Autodesk Inventor part; units mm, degrees
(part 3 of 9)
sketch "Sketch24" plane through (0, 0, 0) normal (1, 0, 0) x (0, 0, -1)
  circle A0 centre (-187.1176, -166.8269) radius 2.4892 projected
  circle A1 centre (-174.2102, -166.8866) radius 2.4892 projected
  circle A2 centre (-167.2175, -120.5501) radius 2.4892 projected
  circle A3 centre (-180.1195, -116.9252) radius 2.4892 projected
  circle A4 centre (-193.0957, -120.1058) radius 2.4892 projected
  circle A5 centre (-186.8225, -117.6771) radius 2.4892 projected
  circle A6 centre (-173.4354, -117.9041) radius 2.4892 projected
  circle A7 centre (-168.1768, -164.3742) radius 2.4892 projected
  circle A8 centre (-180.6733, -167.7222) radius 2.4892 projected
  circle A9 centre (-193.0957, -164.2646) radius 2.4892 projected
  circle A10 centre (0, 0) radius 13.335 projected
  circle A11 centre (160.7915, -118.9794) radius 2.5527 projected
  line L0 (182.8723, -109.8807) -> (181.7836, -109.2266) projected
  arc A12 (170.0112, -99.2275) -> (190.7761, 48.5222) centre (0, 0) ccw projected
  line L1 (204.8485, 54.889) -> (206.0753, 55.2177) projected
  arc A13 (175.4872, -102.4426) -> (196.9261, 50.1033) centre (0, 0) ccw projected
  arc A14 (159.1231, -92.6879) -> (178.5072, 45.237) centre (0, 0) ccw projected
  line L2 (180.312, 48.3145) -> (181.5388, 48.6432) projected
  arc A15 (164.6013, -95.8992) -> (184.6584, 46.8139) centre (0, 0) ccw projected
  line L3 (161.0985, -96.7977) -> (160.0098, -96.1436) projected
  arc A16 (180.8991, -105.7674) -> (203.0448, 51.8076) centre (0, 0) ccw projected
  line L4 (192.5803, 51.6017) -> (193.8071, 51.9305) projected
  arc A17 (186.3731, -108.9857) -> (209.1938, 53.3924) centre (0, 0) ccw projected
  line L5 (171.9854, -103.3393) -> (170.8967, -102.6851) projected
  circle A18 centre (239.2356, -31.496) radius 3.3782 projected
  circle A19 centre (223.7295, 90.3926) radius 3.3782 projected
  circle A20 centre (239.2356, 31.496) radius 3.3782 projected
  circle A21 centre (221.404, -95.9477) radius 3.3782 projected
  line L6 (-35.2916, -50.8) -> (42.0514, -50.8) projected
  arc A22 (74.705, -62.6849) -> (42.0514, -50.8) centre (42.0514, -101.6) ccw projected
  line L7 (74.705, -62.6849) -> (143.4787, -120.3929) projected
  arc A23 (143.8351, -124.9069) -> (143.4787, -120.3929) centre (141.4378, -122.8251) ccw projected
  arc A24 (141.8978, -127.1034) -> (143.8351, -124.9069) centre (0, 0) ccw projected
  arc A25 (141.8978, -127.1034) -> (141.494, -128.2246) centre (143.0803, -128.1626) ccw projected
  line L8 (141.6194, -131.4328) -> (141.494, -128.2246) projected
  arc A26 (141.6194, -131.4328) -> (142.123, -132.5318) centre (143.2057, -131.3708) ccw projected
  line L9 (142.123, -132.5318) -> (176.2311, -164.3381) projected
  arc A27 (176.2311, -164.3381) -> (194.6236, -163.2104) centre (184.8924, -155.0499) ccw projected
  arc A28 (194.6236, -163.2104) -> (235.5329, 95.0804) centre (0, 0) ccw projected
  arc A29 (235.5329, 95.0804) -> (218.389, 101.8364) centre (223.7562, 90.3263) ccw projected
  line L10 (218.389, 101.8364) -> (173.6183, 80.9596) projected
  arc A30 (152.1493, 76.2) -> (173.6183, 80.9596) centre (152.1493, 127) ccw projected
  line L11 (152.1493, 76.2) -> (-101.6, 76.2) projected
  line L12 (-101.6, 76.2) -> (-199.482, -21.682) projected
  line L13 (-199.482, -21.682) -> (-199.482, -255.599) projected
  line L14 (-199.482, -255.599) -> (-35.2916, -255.599) projected
  line L15 (-35.2916, -255.599) -> (-35.2916, -50.8) projected
  line L16 (149.831, -89.2272) -> (89.9434, -38.9755) projected
  line L17 (88.9, -36.7379) -> (88.9, -15.621) projected
  line L18 (91.821, -12.7) -> (174.1799, -12.7) projected
  arc A31 (154.2425, -88.4425) -> (177.0893, -15.8819) centre (0, 0) ccw projected
  line L19 (88.9, -0.254) -> (88.9, 0.254) projected
  line L20 (91.821, 3.175) -> (174.4218, 3.175) projected
  line L21 (177.3428, 0.254) -> (177.3428, -0.254) projected
  line L22 (174.4218, -3.175) -> (91.821, -3.175) projected
  arc A32 (177.0893, 15.8819) -> (169.6939, 53.0738) centre (0, 0) ccw projected
  line L23 (174.1799, 12.7) -> (91.821, 12.7) projected
  line L24 (88.9, 15.621) -> (88.9, 17.1891) projected
  line L25 (90.5865, 19.8364) -> (165.6716, 54.8492) projected
  circle A33 centre (-80.2428, -88.2574) radius 2.4892 projected
  circle A34 centre (-101.8395, -100.8579) radius 2.4892 projected
  circle A35 centre (-93.0185, -51.5569) radius 2.4892 projected
  circle A36 centre (-93.2858, -99.3592) radius 2.4892 projected
  circle A37 centre (-110.6604, -51.6228) radius 2.4892 projected
  circle A38 centre (-124.2369, -62.8574) radius 2.4892 projected
  circle A39 centre (-101.8395, -50.0579) radius 2.4892 projected
  circle A40 centre (-110.3931, -99.2933) radius 2.4892 projected
  circle A41 centre (-85.7798, -94.9817) radius 2.4892 projected
  arc A42 (174.1799, 12.7) -> (177.0893, 15.8819) centre (174.1799, 15.621) ccw projected
  arc A43 (88.9, 15.621) -> (91.821, 12.7) centre (91.821, 15.621) ccw projected
  arc A44 (90.5865, 19.8364) -> (88.9, 17.1891) centre (91.821, 17.1891) ccw projected
  arc A45 (169.6939, 53.0738) -> (165.6716, 54.8492) centre (166.9061, 52.2019) ccw projected
  arc A46 (91.821, 3.175) -> (88.9, 0.254) centre (91.821, 0.254) ccw projected
  arc A47 (177.3428, 0.254) -> (174.4218, 3.175) centre (174.4218, 0.254) ccw projected
  arc A48 (174.4218, -3.175) -> (177.3428, -0.254) centre (174.4218, -0.254) ccw projected
  arc A49 (88.9, -0.254) -> (91.821, -3.175) centre (91.821, -0.254) ccw projected
  arc A50 (88.9, -36.7379) -> (89.9434, -38.9755) centre (91.821, -36.7379) ccw projected
  arc A51 (91.821, -12.7) -> (88.9, -15.621) centre (91.821, -15.621) ccw projected
  arc A52 (177.0893, -15.8819) -> (174.1799, -12.7) centre (174.1799, -15.621) ccw projected
  arc A53 (149.831, -89.2272) -> (154.2425, -88.4425) centre (151.7086, -86.9895) ccw projected
  arc A54 (170.0112, -99.2275) -> (170.8967, -102.6851) centre (172.2049, -100.5079) ccw projected
  arc A55 (192.5803, 51.6017) -> (190.7761, 48.5222) centre (193.2377, 49.1483) ccw projected
  arc A56 (196.9261, 50.1033) -> (193.8071, 51.9305) centre (194.4645, 49.477) ccw projected
  arc A57 (171.9854, -103.3393) -> (175.4872, -102.4426) centre (173.2936, -101.1621) ccw projected
  arc A58 (180.312, 48.3145) -> (178.5072, 45.237) centre (180.9694, 45.861) ccw projected
  arc A59 (184.6584, 46.8139) -> (181.5388, 48.6432) centre (182.1962, 46.1897) ccw projected
  arc A60 (161.0985, -96.7977) -> (164.6013, -95.8992) centre (162.4067, -94.6205) ccw projected
  arc A61 (159.1231, -92.6879) -> (160.0098, -96.1436) centre (161.3179, -93.9664) ccw projected
  arc A62 (204.8485, 54.889) -> (203.0448, 51.8076) centre (205.5059, 52.4355) ccw projected
  arc A63 (209.1938, 53.3924) -> (206.0753, 55.2177) centre (206.7327, 52.7643) ccw projected
  arc A64 (182.8723, -109.8807) -> (186.3731, -108.9857) centre (184.1805, -107.7035) ccw projected
  arc A65 (180.8991, -105.7674) -> (181.7836, -109.2266) centre (183.0918, -107.0494) ccw projected
  arc A66 (-99.6119, -84.758) -> (-99.4903, -84.728) centre (-101.8395, -75.4579) ccw projected
  arc A67 (-99.4903, -84.728) -> (-104.0551, -66.155) centre (-101.7058, -75.4251) ccw projected
  arc A68 (-99.7334, -84.7881) -> (-99.6119, -84.758) centre (-101.9731, -75.491) ccw projected
  arc A69 (-99.8547, -84.8183) -> (-99.7334, -84.7881) centre (-102.1066, -75.5241) ccw projected
  arc A70 (-104.4917, -66.2632) -> (-99.8547, -84.8183) centre (-102.2399, -75.5574) ccw projected
  arc A71 (-104.3463, -66.227) -> (-104.4917, -66.2632) centre (-102.1066, -75.5241) ccw projected
  arc A72 (-104.2008, -66.1909) -> (-104.3463, -66.227) centre (-101.9731, -75.491) ccw projected
  arc A73 (-104.0551, -66.155) -> (-104.2008, -66.1909) centre (-101.8395, -75.4579) ccw projected
  circle A74 centre (0, 0) radius 14.2875
  circle A75 centre (-101.8395, -75.4579) radius 31.75
  line L26 (-136.6187, 12.3445) -> (-98.9084, -11.187)
  line L27 (-98.9084, -11.187) -> (-75.3768, 26.5234)
  line L28 (-75.3768, 26.5234) -> (-113.0872, 50.0549)
  line L29 (-113.0872, 50.0549) -> (-136.6187, 12.3445)
  line L30 (-136.6187, 12.3445) -> (-75.3768, 26.5234) construction
  line L31 (-98.9084, -11.187) -> (-113.0872, 50.0549) construction
  circle A76 centre (-101.8395, -75.4579) radius 44.565
  circle A77 centre (0, 0) radius 15.915
  line L32 (-119.5903, -34.5807) -> (-6.3391, 14.598)
  line L33 (-67.9013, -104.3411) -> (12.12, -10.3147)
  circle A78 centre (0, 0) radius 47.752
  line L34 (-107.8805, 35.2378) -> (-5.6488, 47.4167)
  circle A79 centre (-105.9978, 19.434) radius 15.9156
  line L35 (-113.3646, 5.3259) -> (-22.1029, -42.3286)
  line L36 (-100.8386, 14.2238) -> (-107.9303, 12.3609)
  line L37 (-107.9303, 12.3609) -> (-113.0895, 17.571)
  line L38 (-113.0895, 17.571) -> (-111.157, 24.6441)
  line L39 (-111.157, 24.6441) -> (-104.0652, 26.507)
  line L40 (-104.0652, 26.507) -> (-98.906, 21.2969)
  line L41 (-98.906, 21.2969) -> (-100.8386, 14.2238)
  circle A80 centre (-105.9978, 19.434) radius 7.3323
  circle A81 centre (-101.8395, -75.4579) radius 9.5631
  circle A82 centre (-105.9978, 19.434) radius 9.5631
  circle A83 centre (-101.8395, -75.4579) radius 25.4
  circle A84 centre (-105.9978, 19.434) radius 25.4
  line L42 (-101.8395, -75.4579) -> (0, 0)
  circle A85 centre (0, 0) radius 50.8
  circle A86 centre (-105.9978, 19.434) radius 31.4309
  arc A87 (136.2027, -114.2876) -> (161.1415, 75.1415) centre (0, 0) ccw
  line L43 (0, 0) -> (136.2027, -114.2876)
  line L44 (0, 0) -> (146.4464, 0)
  circle A88 centre (33.8645, -135.5333) radius 88.9
  circle A89 centre (-76.4174, -178.6042) radius 25.4
  line L45 (-88.4199, -21.0451) -> (-93.4785, -9.396)
  circle A90 centre (-76.4174, -178.6042) radius 21.4859
  line L46 (-141.7593, -95.2683) -> (-95.6637, -188.1553)
  line L47 (-57.286, -74.4485) -> (-54.9371, -178.1175)
  line L48 (136.2027, -114.2876) -> (90.5518, -239.7125)
  circle A91 centre (31.6927, -141.5004) radius 88.9
  line L49 (-52.5492, -187.2916) -> (90.6599, -239.4154)
  line L50 (-105.9978, 19.434) -> (0, 0)
  line L51 (-76.4174, -204.0042) -> (-76.4174, -178.6042)
  line L52 (136.2027, -114.2876) -> (136.2027, -239.7125)
  line L53 (-58.8554, 19.434) -> (-105.9978, 19.434)
  circle A92 centre (-17.4502, -276.5193) radius 88.9
  line L54 (-501.4434, -455.6125) -> (248.5176, -455.6125)
  line L55 (-550.7161, -581.025) -> (328.0098, -581.025)
  circle A93 centre (-54.61, -366.7125) radius 88.9
  line L56 (-54.61, -280.9875) -> (-16.51, -280.9875)
  line L57 (-16.51, -280.9875) -> (-16.51, -363.5375)
  line L58 (-16.51, -363.5375) -> (-54.61, -363.5375)
  line L59 (-54.61, -363.5375) -> (-54.61, -280.9875)
  line L60 (-54.61, -322.2625) -> (-16.51, -322.2625)
  line L61 (-54.61, -366.7125) -> (-54.61, -277.8125)
  circle A94 centre (-16.51, -277.8125) radius 88.9
  line L62 (-16.51, -277.8125) -> (-16.51, -366.7125)
  circle A95 centre (-180.2765, -142.3655) radius 31.75
  circle A96 centre (-180.2765, -142.3655) radius 25.4
  circle A97 centre (-180.2765, -142.3655) radius 44.563
  circle A98 centre (-180.2765, -142.3655) radius 9.5631
  line L63 (-194.9575, -184.4408) -> (-91.0984, -220.6795)
  line L64 (-165.5955, -100.2902) -> (-61.7364, -136.5289)
  circle A99 centre (-76.4174, -178.6042) radius 44.563
  line L65 (-167.0299, -113.5109) -> (-119.1112, -9.1307)
  line L66 (-156.1209, -121.7605) -> (-135.7449, -104.3796)
  circle A100 centre (29.8359, -136.4768) radius 88.9
  line L67 (-116.4833, -117.4265) -> (-112.2994, -105.4355)
  point P0 (-35.56, -322.2625)
  dimension "d735" = 63.5
  dimension "d734" = 28.575
  dimension "d736" = 44.45
  dimension "d737" = 31.83
  dimension "d738" = 89.13
  dimension "d739" = 95.504
  dimension "d740" = 31.8313
  dimension "d741" = 12.7
  dimension "d742" = 19.1262
  dimension "d743" = 19.1262
  dimension "d744" = 50.8
  dimension "d745" = 50.8
  dimension "d746" = 107.7646
  dimension "d747" = 126.7485
  dimension "d748" = 101.6
  dimension "d749" = 127
  dimension "d750" = 40
  dimension "d751" = 177.8
  dimension "d752" = 50.8
  dimension "d753" = 12.7
  dimension "d754" = 6.35
  dimension "d755" = 106.233
  dimension "d756" = 152.4
  dimension "d757" = 279.1458
  dimension "d758" = 25
  dimension "d759" = 20
  dimension "d760" = 47.1424
  dimension "d761" = 42.9717
  dimension "d762" = 125.4125
  dimension "d763" = 656.1665
  dimension "d764" = 82.55
  dimension "d765" = 38.1
  dimension "d766" = 1.5989
  dimension "d767" = 35.56
  dimension "d768" = 215.9
  dimension "d769" = 215.9
  dimension "d770" = 26.7819
  dimension "d771" = 114.8539
  dimension "d772" = 109.9998
  dimension "d773" = 581.025
  dimension "d774" = 455.6125
  dimension "d775" = 12.7
  dimension "d776" = 89.1261
  constraints: 84 end point, 26 point on circle, 24 tangent, 23 centre point, 19 coincident, 9 midpoint, 7 perpendicular, 6 equal radius, 6 horizontal, 6 line through centre, 6 point on line, 4 parallel, 4 vertical, 3 concentric, 2 vertical alignment, 26 other
  measures "d734" diameter of A74
  measures "d736" distance of L31.start L28.start
  measures "d737" diameter of A77
  measures "d738" diameter of A76
  measures "d739" diameter of A78
  measures "d740" diameter of A79
  measures "d741" distance between parallel lines of L40 L37
  measures "d742" diameter of A81
  measures "d743" diameter of A82
  measures "d744" diameter of A83
  measures "d745" diameter of A84
  measures "d746" distance of A74.centre point (-105.998, 19.434)
  measures "d747" distance of point (0, 0) point (-101.84, -75.458)
  measures "d748" diameter of A85
  measures "d749" radial gap between concentric circles of A87 A85
  measures "d750" angle of L44 L43
  measures "d751" diameter of A88
  measures "d752" diameter of A89
  measures "d753" distance of L45.start L45.end
  measures "d754" distance of A91.centre A88.centre
  measures "d755" distance of point (-101.84, -75.458) A89.centre
  measures "d756" distance of L49.start L49.end
  measures "d757" vertical distance of L51.start A87.end
  measures "d759" angle of L52 L48
  measures "d760" distance of point (-105.998, 19.434) L53.start
  measures "d761" diameter of A90
  measures "d762" distance between parallel lines of L54 L55
  measures "d763" distance from line of A87.end L55
  measures "d764" distance of L59.start L56.start
  measures "d765" distance of L58.start L59.start
  measures "d766" distance of L62.start A92.centre
  measures "d767" horizontal distance of A85.centre point (-35.56, -322.262)
  measures "d768" distance from line of L54 L52.end
  measures "d769" distance from line of L54 L48.end
  measures "d770" distance of L66.start L66.end
  measures "d771" distance of L65.start L65.end
  measures "d772" distance of A95.centre L51.end
  measures "d773" distance from line of L55 point (0, 0)
  measures "d774" distance from line of L54 L43.start
  measures "d775" distance of L67.start L67.end
  measures "d776" diameter of A97
hole "Pre-Flywheel Bearing Hole" at (0, -178.6042, 76.4174) direction (-1, 0, 0) diameter 26.67 end through all
sketch "Sketch25" plane through (0, 0, 0) normal (1, 0, 0) x (0, 0, -1)
  circle A0 centre (-187.1176, -166.8269) radius 2.4892 projected
  circle A1 centre (-174.2102, -166.8866) radius 2.4892 projected
  circle A2 centre (-167.2175, -120.5501) radius 2.4892 projected
  circle A3 centre (-180.1195, -116.9252) radius 2.4892 projected
  circle A4 centre (-193.0957, -120.1058) radius 2.4892 projected
  circle A5 centre (-186.8225, -117.6771) radius 2.4892 projected
  circle A6 centre (-173.4354, -117.9041) radius 2.4892 projected
  circle A7 centre (-168.1768, -164.3742) radius 2.4892 projected
  circle A8 centre (-180.6733, -167.7222) radius 2.4892 projected
  circle A9 centre (-193.0957, -164.2646) radius 2.4892 projected
  circle A10 centre (0, 0) radius 13.335 projected
  circle A11 centre (160.7915, -118.9794) radius 2.5527 projected
  line L0 (182.8723, -109.8807) -> (181.7836, -109.2266) projected
  arc A12 (170.0112, -99.2275) -> (190.7761, 48.5222) centre (0, 0) ccw projected
  line L1 (204.8485, 54.889) -> (206.0753, 55.2177) projected
  arc A13 (175.4872, -102.4426) -> (196.9261, 50.1033) centre (0, 0) ccw projected
  arc A14 (159.1231, -92.6879) -> (178.5072, 45.237) centre (0, 0) ccw projected
  line L2 (180.312, 48.3145) -> (181.5388, 48.6432) projected
  arc A15 (164.6013, -95.8992) -> (184.6584, 46.8139) centre (0, 0) ccw projected
  line L3 (161.0985, -96.7977) -> (160.0098, -96.1436) projected
  arc A16 (180.8991, -105.7674) -> (203.0448, 51.8076) centre (0, 0) ccw projected
  line L4 (192.5803, 51.6017) -> (193.8071, 51.9305) projected
  arc A17 (186.3731, -108.9857) -> (209.1938, 53.3924) centre (0, 0) ccw projected
  line L5 (171.9854, -103.3393) -> (170.8967, -102.6851) projected
  circle A18 centre (239.2356, -31.496) radius 3.3782 projected
  circle A19 centre (223.7295, 90.3926) radius 3.3782 projected
  circle A20 centre (239.2356, 31.496) radius 3.3782 projected
  circle A21 centre (221.404, -95.9477) radius 3.3782 projected
  line L6 (-35.2916, -50.8) -> (42.0514, -50.8) projected
  arc A22 (74.705, -62.6849) -> (42.0514, -50.8) centre (42.0514, -101.6) ccw projected
  line L7 (74.705, -62.6849) -> (143.4787, -120.3929) projected
  arc A23 (143.8351, -124.9069) -> (143.4787, -120.3929) centre (141.4378, -122.8251) ccw projected
  arc A24 (141.8978, -127.1034) -> (143.8351, -124.9069) centre (0, 0) ccw projected
  arc A25 (141.8978, -127.1034) -> (141.494, -128.2246) centre (143.0803, -128.1626) ccw projected
  line L8 (141.6194, -131.4328) -> (141.494, -128.2246) projected
  arc A26 (141.6194, -131.4328) -> (142.123, -132.5318) centre (143.2057, -131.3708) ccw projected
  line L9 (142.123, -132.5318) -> (176.2311, -164.3381) projected
  arc A27 (176.2311, -164.3381) -> (194.6236, -163.2104) centre (184.8924, -155.0499) ccw projected
  arc A28 (194.6236, -163.2104) -> (235.5329, 95.0804) centre (0, 0) ccw projected
  arc A29 (235.5329, 95.0804) -> (218.389, 101.8364) centre (223.7562, 90.3263) ccw projected
  line L10 (218.389, 101.8364) -> (173.6183, 80.9596) projected
  arc A30 (152.1493, 76.2) -> (173.6183, 80.9596) centre (152.1493, 127) ccw projected
  line L11 (152.1493, 76.2) -> (-101.6, 76.2) projected
  line L12 (-101.6, 76.2) -> (-199.482, -21.682) projected
  line L13 (-199.482, -21.682) -> (-199.482, -255.599) projected
  line L14 (-199.482, -255.599) -> (-35.2916, -255.599) projected
  line L15 (-35.2916, -255.599) -> (-35.2916, -50.8) projected
  line L16 (149.831, -89.2272) -> (89.9434, -38.9755) projected
  line L17 (88.9, -36.7379) -> (88.9, -15.621) projected
  line L18 (91.821, -12.7) -> (174.1799, -12.7) projected
  arc A31 (154.2425, -88.4425) -> (177.0893, -15.8819) centre (0, 0) ccw projected
  line L19 (88.9, -0.254) -> (88.9, 0.254) projected
  line L20 (91.821, 3.175) -> (174.4218, 3.175) projected
  line L21 (177.3428, 0.254) -> (177.3428, -0.254) projected
  line L22 (174.4218, -3.175) -> (91.821, -3.175) projected
  arc A32 (177.0893, 15.8819) -> (169.6939, 53.0738) centre (0, 0) ccw projected
  line L23 (174.1799, 12.7) -> (91.821, 12.7) projected
  line L24 (88.9, 15.621) -> (88.9, 17.1891) projected
  line L25 (90.5865, 19.8364) -> (165.6716, 54.8492) projected
  circle A33 centre (-80.2428, -88.2574) radius 2.4892 projected
  circle A34 centre (-101.8395, -100.8579) radius 2.4892 projected
  circle A35 centre (-93.0185, -51.5569) radius 2.4892 projected
  circle A36 centre (-93.2858, -99.3592) radius 2.4892 projected
  circle A37 centre (-110.6604, -51.6228) radius 2.4892 projected
  circle A38 centre (-124.2369, -62.8574) radius 2.4892 projected
  circle A39 centre (-101.8395, -50.0579) radius 2.4892 projected
  circle A40 centre (-110.3931, -99.2933) radius 2.4892 projected
  circle A41 centre (-85.7798, -94.9817) radius 2.4892 projected
  arc A42 (174.1799, 12.7) -> (177.0893, 15.8819) centre (174.1799, 15.621) ccw projected
  arc A43 (88.9, 15.621) -> (91.821, 12.7) centre (91.821, 15.621) ccw projected
  arc A44 (90.5865, 19.8364) -> (88.9, 17.1891) centre (91.821, 17.1891) ccw projected
  arc A45 (169.6939, 53.0738) -> (165.6716, 54.8492) centre (166.9061, 52.2019) ccw projected
  arc A46 (91.821, 3.175) -> (88.9, 0.254) centre (91.821, 0.254) ccw projected
  arc A47 (177.3428, 0.254) -> (174.4218, 3.175) centre (174.4218, 0.254) ccw projected
  arc A48 (174.4218, -3.175) -> (177.3428, -0.254) centre (174.4218, -0.254) ccw projected
  arc A49 (88.9, -0.254) -> (91.821, -3.175) centre (91.821, -0.254) ccw projected
  arc A50 (88.9, -36.7379) -> (89.9434, -38.9755) centre (91.821, -36.7379) ccw projected
  arc A51 (91.821, -12.7) -> (88.9, -15.621) centre (91.821, -15.621) ccw projected
  arc A52 (177.0893, -15.8819) -> (174.1799, -12.7) centre (174.1799, -15.621) ccw projected
  arc A53 (149.831, -89.2272) -> (154.2425, -88.4425) centre (151.7086, -86.9895) ccw projected
  arc A54 (170.0112, -99.2275) -> (170.8967, -102.6851) centre (172.2049, -100.5079) ccw projected
  arc A55 (192.5803, 51.6017) -> (190.7761, 48.5222) centre (193.2377, 49.1483) ccw projected
  arc A56 (196.9261, 50.1033) -> (193.8071, 51.9305) centre (194.4645, 49.477) ccw projected
  arc A57 (171.9854, -103.3393) -> (175.4872, -102.4426) centre (173.2936, -101.1621) ccw projected
  arc A58 (180.312, 48.3145) -> (178.5072, 45.237) centre (180.9694, 45.861) ccw projected
  arc A59 (184.6584, 46.8139) -> (181.5388, 48.6432) centre (182.1962, 46.1897) ccw projected
  arc A60 (161.0985, -96.7977) -> (164.6013, -95.8992) centre (162.4067, -94.6205) ccw projected
  arc A61 (159.1231, -92.6879) -> (160.0098, -96.1436) centre (161.3179, -93.9664) ccw projected
  arc A62 (204.8485, 54.889) -> (203.0448, 51.8076) centre (205.5059, 52.4355) ccw projected
  arc A63 (209.1938, 53.3924) -> (206.0753, 55.2177) centre (206.7327, 52.7643) ccw projected
  arc A64 (182.8723, -109.8807) -> (186.3731, -108.9857) centre (184.1805, -107.7035) ccw projected
  arc A65 (180.8991, -105.7674) -> (181.7836, -109.2266) centre (183.0918, -107.0494) ccw projected
  arc A66 (-99.6119, -84.758) -> (-99.4903, -84.728) centre (-101.8395, -75.4579) ccw projected
  arc A67 (-99.4903, -84.728) -> (-104.0551, -66.155) centre (-101.7058, -75.4251) ccw projected
  arc A68 (-99.7334, -84.7881) -> (-99.6119, -84.758) centre (-101.9731, -75.491) ccw projected
  arc A69 (-99.8547, -84.8183) -> (-99.7334, -84.7881) centre (-102.1066, -75.5241) ccw projected
  arc A70 (-104.4917, -66.2632) -> (-99.8547, -84.8183) centre (-102.2399, -75.5574) ccw projected
  arc A71 (-104.3463, -66.227) -> (-104.4917, -66.2632) centre (-102.1066, -75.5241) ccw projected
  arc A72 (-104.2008, -66.1909) -> (-104.3463, -66.227) centre (-101.9731, -75.491) ccw projected
  arc A73 (-104.0551, -66.155) -> (-104.2008, -66.1909) centre (-101.8395, -75.4579) ccw projected
  circle A74 centre (-76.4174, -178.6042) radius 13.335 projected
  circle A75 centre (-187.1176, -166.8269) radius 2.4892 projected
  circle A76 centre (-174.2102, -166.8866) radius 2.4892 projected
  circle A77 centre (-167.2175, -120.5501) radius 2.4892 projected
  circle A78 centre (-180.1195, -116.9252) radius 2.4892 projected
  circle A79 centre (-193.0957, -120.1058) radius 2.4892 projected
  circle A80 centre (-186.8225, -117.6771) radius 2.4892 projected
  circle A81 centre (-173.4354, -117.9041) radius 2.4892 projected
  circle A82 centre (-168.1768, -164.3742) radius 2.4892 projected
  circle A83 centre (-180.6733, -167.7222) radius 2.4892 projected
  circle A84 centre (-193.0957, -164.2646) radius 2.4892 projected
  arc A85 (-183.7267, -151.29) -> (-183.6068, -151.3318) centre (-180.5163, -142.2818) ccw projected
  arc A86 (-177.4258, -133.2319) -> (-183.7267, -151.29) centre (-180.6362, -142.24) ccw projected
  arc A87 (-177.3059, -133.2737) -> (-177.4258, -133.2319) centre (-180.5163, -142.2818) ccw projected
  arc A88 (-177.186, -133.3155) -> (-177.3059, -133.2737) centre (-180.3964, -142.3237) ccw projected
  arc A89 (-177.0661, -133.3574) -> (-177.186, -133.3155) centre (-180.2765, -142.3655) ccw projected
  arc A90 (-183.367, -151.4155) -> (-177.0661, -133.3574) centre (-180.1566, -142.4074) ccw projected
  arc A91 (-183.4869, -151.3736) -> (-183.367, -151.4155) centre (-180.2765, -142.3655) ccw projected
  arc A92 (-183.6068, -151.3318) -> (-183.4869, -151.3736) centre (-180.3964, -142.3237) ccw projected
  circle A93 centre (-85.7798, -94.9817) radius 2.4892 projected
  circle A94 centre (-110.3931, -99.2933) radius 2.4892 projected
  circle A95 centre (-101.8395, -50.0579) radius 2.4892 projected
  circle A96 centre (-124.2369, -62.8574) radius 2.4892 projected
  circle A97 centre (-110.6604, -51.6228) radius 2.4892 projected
  circle A98 centre (-93.2858, -99.3592) radius 2.4892 projected
  circle A99 centre (-118.4334, -56.0666) radius 2.4892 projected
  circle A100 centre (-93.0185, -51.5569) radius 2.4892 projected
  circle A101 centre (-101.8395, -100.8579) radius 2.4892 projected
  circle A102 centre (-80.2428, -88.2574) radius 2.4892 projected
  arc A103 (-99.4903, -84.728) -> (-104.0551, -66.155) centre (-101.7058, -75.4251) ccw projected
  arc A104 (-99.6119, -84.758) -> (-99.4903, -84.728) centre (-101.8395, -75.4579) ccw projected
  arc A105 (-99.7334, -84.7881) -> (-99.6119, -84.758) centre (-101.9731, -75.491) ccw projected
  arc A106 (-99.8547, -84.8183) -> (-99.7334, -84.7881) centre (-102.1066, -75.5241) ccw projected
  arc A107 (-104.4917, -66.2632) -> (-99.8547, -84.8183) centre (-102.2399, -75.5574) ccw projected
  arc A108 (-104.3463, -66.227) -> (-104.4917, -66.2632) centre (-102.1066, -75.5241) ccw projected
  arc A109 (-104.2008, -66.1909) -> (-104.3463, -66.227) centre (-101.9731, -75.491) ccw projected
  arc A110 (-104.0551, -66.155) -> (-104.2008, -66.1909) centre (-101.8395, -75.4579) ccw projected
  circle A111 centre (239.2356, -31.496) radius 3.3782 projected
  circle A112 centre (223.7295, 90.3926) radius 3.3782 projected
  circle A113 centre (239.2356, 31.496) radius 3.3782 projected
  circle A114 centre (221.404, -95.9477) radius 3.3782 projected
  line L26 (-35.2916, -50.8) -> (42.0514, -50.8) projected
  arc A115 (74.705, -62.6849) -> (42.0514, -50.8) centre (42.0514, -101.6) ccw projected
  line L27 (74.705, -62.6849) -> (143.4787, -120.3929) projected
  arc A116 (143.8351, -124.9069) -> (143.4787, -120.3929) centre (141.4378, -122.8251) ccw projected
  arc A117 (141.8978, -127.1034) -> (143.8351, -124.9069) centre (0, 0) ccw projected
  arc A118 (141.8978, -127.1034) -> (141.494, -128.2246) centre (143.0803, -128.1626) ccw projected
  line L28 (141.6194, -131.4328) -> (141.494, -128.2246) projected
  arc A119 (141.6194, -131.4328) -> (142.123, -132.5318) centre (143.2057, -131.3708) ccw projected
  line L29 (142.123, -132.5318) -> (176.2311, -164.3381) projected
  arc A120 (176.2311, -164.3381) -> (194.6236, -163.2104) centre (184.8924, -155.0499) ccw projected
  arc A121 (194.6236, -163.2104) -> (235.5329, 95.0804) centre (0, 0) ccw projected
  arc A122 (235.5329, 95.0804) -> (218.389, 101.8364) centre (223.7562, 90.3263) ccw projected
  line L30 (218.389, 101.8364) -> (173.6183, 80.9596) projected
  arc A123 (152.1493, 76.2) -> (173.6183, 80.9596) centre (152.1493, 127) ccw projected
  line L31 (152.1493, 76.2) -> (-101.6, 76.2) projected
  line L32 (-101.6, 76.2) -> (-199.482, -21.682) projected
  line L33 (-199.482, -21.682) -> (-199.482, -255.599) projected
  line L34 (-199.482, -255.599) -> (-35.2916, -255.599) projected
  line L35 (-35.2916, -255.599) -> (-35.2916, -50.8) projected
  line L36 (149.831, -89.2272) -> (89.9434, -38.9755) projected
  arc A124 (88.9, -36.7379) -> (89.9434, -38.9755) centre (91.821, -36.7379) ccw projected
  line L37 (88.9, -36.7379) -> (88.9, -15.621) projected
  arc A125 (91.821, -12.7) -> (88.9, -15.621) centre (91.821, -15.621) ccw projected
  line L38 (91.821, -12.7) -> (174.1799, -12.7) projected
  arc A126 (177.0893, -15.8819) -> (174.1799, -12.7) centre (174.1799, -15.621) ccw projected
  arc A127 (154.2425, -88.4425) -> (177.0893, -15.8819) centre (0, 0) ccw projected
  arc A128 (149.831, -89.2272) -> (154.2425, -88.4425) centre (151.7086, -86.9895) ccw projected
  line L39 (88.9, -0.254) -> (88.9, 0.254) projected
  arc A129 (91.821, 3.175) -> (88.9, 0.254) centre (91.821, 0.254) ccw projected
  line L40 (91.821, 3.175) -> (174.4218, 3.175) projected
  arc A130 (177.3428, 0.254) -> (174.4218, 3.175) centre (174.4218, 0.254) ccw projected
  line L41 (177.3428, 0.254) -> (177.3428, -0.254) projected
  arc A131 (174.4218, -3.175) -> (177.3428, -0.254) centre (174.4218, -0.254) ccw projected
  line L42 (174.4218, -3.175) -> (91.821, -3.175) projected
  arc A132 (88.9, -0.254) -> (91.821, -3.175) centre (91.821, -0.254) ccw projected
  arc A133 (177.0893, 15.8819) -> (169.6939, 53.0738) centre (0, 0) ccw projected
  arc A134 (174.1799, 12.7) -> (177.0893, 15.8819) centre (174.1799, 15.621) ccw projected
  line L43 (174.1799, 12.7) -> (91.821, 12.7) projected
  arc A135 (88.9, 15.621) -> (91.821, 12.7) centre (91.821, 15.621) ccw projected
  line L44 (88.9, 15.621) -> (88.9, 17.1891) projected
  arc A136 (90.5865, 19.8364) -> (88.9, 17.1891) centre (91.821, 17.1891) ccw projected
  line L45 (90.5865, 19.8364) -> (165.6716, 54.8492) projected
  arc A137 (169.6939, 53.0738) -> (165.6716, 54.8492) centre (166.9061, 52.2019) ccw projected
  arc A138 (180.8991, -105.7674) -> (203.0448, 51.8076) centre (0, 0) ccw projected
  arc A139 (204.8485, 54.889) -> (203.0448, 51.8076) centre (205.5059, 52.4355) ccw projected
  line L46 (204.8485, 54.889) -> (206.0753, 55.2177) projected
  arc A140 (209.1938, 53.3924) -> (206.0753, 55.2177) centre (206.7327, 52.7643) ccw projected
  arc A141 (186.3731, -108.9857) -> (209.1938, 53.3924) centre (0, 0) ccw projected
  arc A142 (182.8723, -109.8807) -> (186.3731, -108.9857) centre (184.1805, -107.7035) ccw projected
  line L47 (182.8723, -109.8807) -> (181.7836, -109.2266) projected
  arc A143 (180.8991, -105.7674) -> (181.7836, -109.2266) centre (183.0918, -107.0494) ccw projected
  arc A144 (159.1231, -92.6879) -> (178.5072, 45.237) centre (0, 0) ccw projected
  arc A145 (180.312, 48.3145) -> (178.5072, 45.237) centre (180.9694, 45.861) ccw projected
  line L48 (180.312, 48.3145) -> (181.5388, 48.6432) projected
  arc A146 (184.6584, 46.8139) -> (181.5388, 48.6432) centre (182.1962, 46.1897) ccw projected
  arc A147 (164.6013, -95.8992) -> (184.6584, 46.8139) centre (0, 0) ccw projected
  arc A148 (161.0985, -96.7977) -> (164.6013, -95.8992) centre (162.4067, -94.6205) ccw projected
  line L49 (161.0985, -96.7977) -> (160.0098, -96.1436) projected
  arc A149 (159.1231, -92.6879) -> (160.0098, -96.1436) centre (161.3179, -93.9664) ccw projected
  line L50 (171.9854, -103.3393) -> (170.8967, -102.6851) projected
  arc A150 (170.0112, -99.2275) -> (170.8967, -102.6851) centre (172.2049, -100.5079) ccw projected
  arc A151 (170.0112, -99.2275) -> (190.7761, 48.5222) centre (0, 0) ccw projected
  arc A152 (192.5803, 51.6017) -> (190.7761, 48.5222) centre (193.2377, 49.1483) ccw projected
  line L51 (192.5803, 51.6017) -> (193.8071, 51.9305) projected
  arc A153 (196.9261, 50.1033) -> (193.8071, 51.9305) centre (194.4645, 49.477) ccw projected
  arc A154 (175.4872, -102.4426) -> (196.9261, 50.1033) centre (0, 0) ccw projected
  arc A155 (171.9854, -103.3393) -> (175.4872, -102.4426) centre (173.2936, -101.1621) ccw projected
  circle A156 centre (187.962, 68.4126) radius 2.5527 projected
  circle A157 centre (160.7915, -118.9794) radius 2.5527 projected
  circle A158 centre (0, 0) radius 13.335 projected
  line L52 (-183.7867, -151.2692) -> (-183.3071, -151.4366)
  line L53 (-183.3071, -151.4366) -> (-177.0061, -133.3781)
  line L54 (-177.0061, -133.3781) -> (-177.4857, -133.2108)
  line L55 (-177.4857, -133.2108) -> (-183.7867, -151.2692)
  arc A159 (-177.4258, -133.2319) -> (-183.7267, -151.29) centre (-180.6362, -142.24) ccw projected
  arc A160 (-183.367, -151.4155) -> (-177.0661, -133.3574) centre (-180.1566, -142.4074) ccw projected
  constraints: 8 end point, 4 tangent, 2 midpoint, 2 parallel, 1 perpendicular
extrude "Extrusion15" cut sketch "Sketch25" against normal through all contours A86 L55 A87 A88 A89 A90 L53 A91 A92 A85
sketch "Sketch26" plane through (0, 0, 0) normal (1, 0, 0) x (0, 0, -1)
  circle A0 centre (-187.1176, -166.8269) radius 2.4892 projected
  circle A1 centre (-174.2102, -166.8866) radius 2.4892 projected
  circle A2 centre (-167.2175, -120.5501) radius 2.4892 projected
  circle A3 centre (-180.1195, -116.9252) radius 2.4892 projected
  circle A4 centre (-193.0957, -120.1058) radius 2.4892 projected
  circle A5 centre (-186.8225, -117.6771) radius 2.4892 projected
  circle A6 centre (-173.4354, -117.9041) radius 2.4892 projected
  circle A7 centre (-168.1768, -164.3742) radius 2.4892 projected
  circle A8 centre (-180.6733, -167.7222) radius 2.4892 projected
  circle A9 centre (-193.0957, -164.2646) radius 2.4892 projected
  circle A10 centre (0, 0) radius 13.335 projected
  circle A11 centre (160.7915, -118.9794) radius 2.5527 projected
  line L0 (182.8723, -109.8807) -> (181.7836, -109.2266) projected
  arc A12 (170.0112, -99.2275) -> (190.7761, 48.5222) centre (0, 0) ccw projected
  line L1 (204.8485, 54.889) -> (206.0753, 55.2177) projected
  arc A13 (175.4872, -102.4426) -> (196.9261, 50.1033) centre (0, 0) ccw projected
  arc A14 (159.1231, -92.6879) -> (178.5072, 45.237) centre (0, 0) ccw projected
  line L2 (180.312, 48.3145) -> (181.5388, 48.6432) projected
  arc A15 (164.6013, -95.8992) -> (184.6584, 46.8139) centre (0, 0) ccw projected
  line L3 (161.0985, -96.7977) -> (160.0098, -96.1436) projected
  arc A16 (180.8991, -105.7674) -> (203.0448, 51.8076) centre (0, 0) ccw projected
  line L4 (192.5803, 51.6017) -> (193.8071, 51.9305) projected
  arc A17 (186.3731, -108.9857) -> (209.1938, 53.3924) centre (0, 0) ccw projected
  line L5 (171.9854, -103.3393) -> (170.8967, -102.6851) projected
  circle A18 centre (239.2356, -31.496) radius 3.3782 projected
  circle A19 centre (223.7295, 90.3926) radius 3.3782 projected
  circle A20 centre (239.2356, 31.496) radius 3.3782 projected
  circle A21 centre (221.404, -95.9477) radius 3.3782 projected
  line L6 (-35.2916, -50.8) -> (42.0514, -50.8) projected
  arc A22 (74.705, -62.6849) -> (42.0514, -50.8) centre (42.0514, -101.6) ccw projected
  line L7 (74.705, -62.6849) -> (143.4787, -120.3929) projected
  arc A23 (143.8351, -124.9069) -> (143.4787, -120.3929) centre (141.4378, -122.8251) ccw projected
  arc A24 (141.8978, -127.1034) -> (143.8351, -124.9069) centre (0, 0) ccw projected
  arc A25 (141.8978, -127.1034) -> (141.494, -128.2246) centre (143.0803, -128.1626) ccw projected
  line L8 (141.6194, -131.4328) -> (141.494, -128.2246) projected
  arc A26 (141.6194, -131.4328) -> (142.123, -132.5318) centre (143.2057, -131.3708) ccw projected
  line L9 (142.123, -132.5318) -> (176.2311, -164.3381) projected
  arc A27 (176.2311, -164.3381) -> (194.6236, -163.2104) centre (184.8924, -155.0499) ccw projected
  arc A28 (194.6236, -163.2104) -> (235.5329, 95.0804) centre (0, 0) ccw projected
  arc A29 (235.5329, 95.0804) -> (218.389, 101.8364) centre (223.7562, 90.3263) ccw projected
  line L10 (218.389, 101.8364) -> (173.6183, 80.9596) projected
  arc A30 (152.1493, 76.2) -> (173.6183, 80.9596) centre (152.1493, 127) ccw projected
  line L11 (152.1493, 76.2) -> (-101.6, 76.2) projected
  line L12 (-101.6, 76.2) -> (-199.482, -21.682) projected
  line L13 (-199.482, -21.682) -> (-199.482, -255.599) projected
  line L14 (-199.482, -255.599) -> (-35.2916, -255.599) projected
  line L15 (-35.2916, -255.599) -> (-35.2916, -50.8) projected
  line L16 (149.831, -89.2272) -> (89.9434, -38.9755) projected
  line L17 (88.9, -36.7379) -> (88.9, -15.621) projected
  line L18 (91.821, -12.7) -> (174.1799, -12.7) projected
  arc A31 (154.2425, -88.4425) -> (177.0893, -15.8819) centre (0, 0) ccw projected
  line L19 (88.9, -0.254) -> (88.9, 0.254) projected
  line L20 (91.821, 3.175) -> (174.4218, 3.175) projected
  line L21 (177.3428, 0.254) -> (177.3428, -0.254) projected
  line L22 (174.4218, -3.175) -> (91.821, -3.175) projected
  arc A32 (177.0893, 15.8819) -> (169.6939, 53.0738) centre (0, 0) ccw projected
  line L23 (174.1799, 12.7) -> (91.821, 12.7) projected
  line L24 (88.9, 15.621) -> (88.9, 17.1891) projected
  line L25 (90.5865, 19.8364) -> (165.6716, 54.8492) projected
  circle A33 centre (-80.2428, -88.2574) radius 2.4892 projected
  circle A34 centre (-101.8395, -100.8579) radius 2.4892 projected
  circle A35 centre (-93.0185, -51.5569) radius 2.4892 projected
  circle A36 centre (-93.2858, -99.3592) radius 2.4892 projected
  circle A37 centre (-110.6604, -51.6228) radius 2.4892 projected
  circle A38 centre (-124.2369, -62.8574) radius 2.4892 projected
  circle A39 centre (-101.8395, -50.0579) radius 2.4892 projected
  circle A40 centre (-110.3931, -99.2933) radius 2.4892 projected
  circle A41 centre (-85.7798, -94.9817) radius 2.4892 projected
  circle A42 centre (-117.3868, 181.1992) radius 9.5631
  line L26 (-58.8554, 19.434) -> (-105.9978, 19.434)
  line L27 (-85.3603, 1.9715) -> (-126.6353, 1.9715)
  line L28 (-126.6353, 1.9715) -> (-126.6353, 36.8965)
  line L29 (-126.6353, 36.8965) -> (-85.3603, 36.8965)
  line L30 (-85.3603, 36.8965) -> (-85.3603, 1.9715)
  line L31 (-85.3603, 1.9715) -> (-126.6353, 36.8965) construction
  line L32 (-126.6353, 1.9715) -> (-85.3603, 36.8965) construction
  line L33 (-132.3503, 19.434) -> (-79.6453, 19.434)
  circle A43 centre (-132.3503, 19.434) radius 3.175
  circle A44 centre (-79.6453, 19.434) radius 3.175
  line L34 (-132.3503, 22.609) -> (-126.6353, 22.609)
  line L35 (-132.3503, 16.259) -> (-126.6353, 16.259)
  line L36 (-85.3603, 22.609) -> (-79.6453, 22.609)
  line L37 (-79.6453, 16.259) -> (-85.3603, 16.259)
  arc A45 (174.1799, 12.7) -> (177.0893, 15.8819) centre (174.1799, 15.621) ccw projected
  arc A46 (88.9, 15.621) -> (91.821, 12.7) centre (91.821, 15.621) ccw projected
  arc A47 (90.5865, 19.8364) -> (88.9, 17.1891) centre (91.821, 17.1891) ccw projected
  arc A48 (169.6939, 53.0738) -> (165.6716, 54.8492) centre (166.9061, 52.2019) ccw projected
  arc A49 (91.821, 3.175) -> (88.9, 0.254) centre (91.821, 0.254) ccw projected
  arc A50 (177.3428, 0.254) -> (174.4218, 3.175) centre (174.4218, 0.254) ccw projected
  arc A51 (174.4218, -3.175) -> (177.3428, -0.254) centre (174.4218, -0.254) ccw projected
  arc A52 (88.9, -0.254) -> (91.821, -3.175) centre (91.821, -0.254) ccw projected
  arc A53 (88.9, -36.7379) -> (89.9434, -38.9755) centre (91.821, -36.7379) ccw projected
  arc A54 (91.821, -12.7) -> (88.9, -15.621) centre (91.821, -15.621) ccw projected
  arc A55 (177.0893, -15.8819) -> (174.1799, -12.7) centre (174.1799, -15.621) ccw projected
  arc A56 (149.831, -89.2272) -> (154.2425, -88.4425) centre (151.7086, -86.9895) ccw projected
  arc A57 (170.0112, -99.2275) -> (170.8967, -102.6851) centre (172.2049, -100.5079) ccw projected
  arc A58 (192.5803, 51.6017) -> (190.7761, 48.5222) centre (193.2377, 49.1483) ccw projected
  arc A59 (196.9261, 50.1033) -> (193.8071, 51.9305) centre (194.4645, 49.477) ccw projected
  arc A60 (171.9854, -103.3393) -> (175.4872, -102.4426) centre (173.2936, -101.1621) ccw projected
  arc A61 (180.312, 48.3145) -> (178.5072, 45.237) centre (180.9694, 45.861) ccw projected
  arc A62 (184.6584, 46.8139) -> (181.5388, 48.6432) centre (182.1962, 46.1897) ccw projected
  arc A63 (161.0985, -96.7977) -> (164.6013, -95.8992) centre (162.4067, -94.6205) ccw projected
  arc A64 (159.1231, -92.6879) -> (160.0098, -96.1436) centre (161.3179, -93.9664) ccw projected
  arc A65 (204.8485, 54.889) -> (203.0448, 51.8076) centre (205.5059, 52.4355) ccw projected
  arc A66 (209.1938, 53.3924) -> (206.0753, 55.2177) centre (206.7327, 52.7643) ccw projected
  arc A67 (182.8723, -109.8807) -> (186.3731, -108.9857) centre (184.1805, -107.7035) ccw projected
  arc A68 (180.8991, -105.7674) -> (181.7836, -109.2266) centre (183.0918, -107.0494) ccw projected
  arc A69 (-99.6119, -84.758) -> (-99.4903, -84.728) centre (-101.8395, -75.4579) ccw projected
  arc A70 (-99.4903, -84.728) -> (-104.0551, -66.155) centre (-101.7058, -75.4251) ccw projected
  arc A71 (-99.7334, -84.7881) -> (-99.6119, -84.758) centre (-101.9731, -75.491) ccw projected
  arc A72 (-99.8547, -84.8183) -> (-99.7334, -84.7881) centre (-102.1066, -75.5241) ccw projected
  arc A73 (-104.4917, -66.2632) -> (-99.8547, -84.8183) centre (-102.2399, -75.5574) ccw projected
  arc A74 (-104.3463, -66.227) -> (-104.4917, -66.2632) centre (-102.1066, -75.5241) ccw projected
  arc A75 (-104.2008, -66.1909) -> (-104.3463, -66.227) centre (-101.9731, -75.491) ccw projected
  arc A76 (-104.0551, -66.155) -> (-104.2008, -66.1909) centre (-101.8395, -75.4579) ccw projected
  circle A77 centre (0, 0) radius 14.2875
  circle A78 centre (-101.8395, -75.4579) radius 31.75
  line L38 (-136.9268, 13.8395) -> (-100.4033, -11.4951)
  line L39 (-100.4033, -11.4951) -> (-75.0688, 25.0284)
  line L40 (-75.0688, 25.0284) -> (-111.5922, 50.363)
  line L41 (-111.5922, 50.363) -> (-136.9268, 13.8395)
  line L42 (-136.9268, 13.8395) -> (-75.0688, 25.0284) construction
  line L43 (-100.4033, -11.4951) -> (-111.5922, 50.363) construction
  circle A79 centre (-101.8395, -75.4579) radius 44.565
  circle A80 centre (0, 0) radius 15.915
  line L44 (-119.5903, -34.5807) -> (-6.3391, 14.598)
  line L45 (-67.9013, -104.3411) -> (12.12, -10.3147)
  circle A81 centre (0, 0) radius 47.752
  line L46 (-107.8805, 35.2378) -> (-5.6488, 47.4167)
  circle A82 centre (-105.9978, 19.434) radius 15.9156
  line L47 (-113.3646, 5.3259) -> (-22.1029, -42.3286)
  line L48 (-101.0714, 14.0031) -> (-108.2378, 12.4522)
  line L49 (-108.2378, 12.4522) -> (-113.1642, 17.883)
  line L50 (-113.1642, 17.883) -> (-110.9242, 24.8648)
  line L51 (-110.9242, 24.8648) -> (-103.7577, 26.4158)
  line L52 (-103.7577, 26.4158) -> (-98.8313, 20.9849)
  line L53 (-98.8313, 20.9849) -> (-101.0714, 14.0031)
  circle A83 centre (-105.9978, 19.434) radius 7.3323
  circle A84 centre (-101.8395, -75.4579) radius 9.5631
  circle A85 centre (-105.9978, 19.434) radius 9.5631
  circle A86 centre (-101.8395, -75.4579) radius 25.4
  circle A87 centre (-105.9978, 19.434) radius 25.4
  line L54 (-101.8395, -75.4579) -> (0, 0)
  circle A88 centre (0, 0) radius 50.8
  circle A89 centre (-105.9978, 19.434) radius 31.4309
  arc A90 (136.2027, -114.2876) -> (161.1415, 75.1415) centre (0, 0) ccw
  line L55 (0, 0) -> (136.2027, -114.2876)
  line L56 (0, 0) -> (159.0178, 0)
  circle A91 centre (33.8645, -135.5333) radius 88.9
  circle A92 centre (-76.4174, -178.6042) radius 25.4
  line L57 (-88.4199, -21.0451) -> (-93.4785, -9.396)
  circle A93 centre (-76.4174, -178.6042) radius 21.4859
  line L58 (-141.7593, -95.2683) -> (-95.6637, -188.1553)
  line L59 (-57.286, -74.4485) -> (-54.9371, -178.1175)
  line L60 (136.2027, -114.2876) -> (90.5518, -239.7125)
  circle A94 centre (31.6927, -141.5004) radius 88.9
  line L61 (-52.5492, -187.2916) -> (90.6599, -239.4154)
  line L62 (-105.9978, 19.434) -> (0, 0)
  line L63 (-76.4174, -204.0042) -> (-76.4174, -178.6042)
  line L64 (136.2027, -114.2876) -> (136.2027, -239.7125)
  line L65 (-58.8554, 19.434) -> (-105.9978, 19.434)
  circle A95 centre (-17.4502, -276.5193) radius 88.9
  line L66 (-501.4434, -455.6125) -> (248.5176, -455.6125)
  line L67 (-550.7161, -581.025) -> (328.0098, -581.025)
  circle A96 centre (-54.61, -366.7125) radius 88.9
  line L68 (-54.61, -280.9875) -> (-16.51, -280.9875)
  line L69 (-16.51, -280.9875) -> (-16.51, -363.5375)
  line L70 (-16.51, -363.5375) -> (-54.61, -363.5375)
  line L71 (-54.61, -363.5375) -> (-54.61, -280.9875)
  line L72 (-54.61, -322.2625) -> (-16.51, -322.2625)
  line L73 (-54.61, -366.7125) -> (-54.61, -277.8125)
  circle A97 centre (-16.51, -277.8125) radius 88.9
  line L74 (-16.51, -277.8125) -> (-16.51, -366.7125)
  circle A98 centre (-180.2765, -142.3655) radius 31.75
  circle A99 centre (-180.2765, -142.3655) radius 25.4
  circle A100 centre (-180.2765, -142.3655) radius 44.563
  circle A101 centre (-180.2765, -142.3655) radius 9.5631
  line L75 (-194.9575, -184.4408) -> (-91.0984, -220.6795)
  line L76 (-165.5955, -100.2902) -> (-61.7364, -136.5289)
  circle A102 centre (-76.4174, -178.6042) radius 44.563
  line L77 (-167.0299, -113.5109) -> (-119.1112, -9.1307)
  line L78 (-156.1209, -121.7605) -> (-135.7449, -104.3796)
  circle A103 centre (29.8359, -136.4768) radius 88.9
  line L79 (-116.4833, -117.4265) -> (-112.2994, -105.4355)
  point P0 (-35.56, -322.2625)
  dimension "d778" = 63.5
  dimension "d392" = 19.1262
  dimension "d409" = 47.1424
  dimension "d422" = 34.925
  dimension "d423" = 41.275
  dimension "d424" = 52.705
  dimension "d425" = 6.35
  dimension "d777" = 28.575
  dimension "d779" = 44.45
  dimension "d780" = 31.83
  dimension "d781" = 89.13
  dimension "d782" = 95.504
  dimension "d783" = 31.8313
  dimension "d784" = 12.7
  dimension "d785" = 19.1262
  dimension "d786" = 19.1262
  dimension "d787" = 50.8
  dimension "d788" = 50.8
  dimension "d789" = 107.7646
  dimension "d790" = 126.7485
  dimension "d791" = 101.6
  dimension "d792" = 127
  dimension "d793" = 40
  dimension "d794" = 177.8
  dimension "d795" = 50.8
  dimension "d796" = 12.7
  dimension "d797" = 6.35
  dimension "d798" = 106.233
  dimension "d799" = 152.4
  dimension "d800" = 279.1458
  dimension "d801" = 25
  dimension "d802" = 20
  dimension "d803" = 47.1424
  dimension "d804" = 42.9717
  dimension "d805" = 125.4125
  dimension "d806" = 656.1665
  dimension "d807" = 82.55
  dimension "d808" = 38.1
  dimension "d809" = 1.5989
  dimension "d810" = 35.56
  dimension "d811" = 215.9
  dimension "d812" = 215.9
  dimension "d813" = 26.7819
  dimension "d814" = 114.8539
  dimension "d815" = 109.9998
  dimension "d816" = 581.025
  dimension "d817" = 455.6125
  dimension "d818" = 12.7
  dimension "d819" = 89.1261
  constraints: 108 end point, 30 point on circle, 28 tangent, 26 centre point, 23 coincident, 12 midpoint, 11 horizontal, 10 perpendicular, 10 point on line, 7 equal radius, 6 line through centre, 6 parallel, 4 vertical, 3 concentric, 2 vertical alignment, 26 other
  measures "d392" diameter of A42
  measures "d409" distance of point (-105.998, 19.434) L26.start
  measures "d422" distance of L27.end L28.end
  measures "d423" distance of L28.end L29.end
  measures "d424" distance of L33.start L33.end
  measures "d425" diameter of A43
  measures "d777" diameter of A77
  measures "d779" distance of L39.start L40.start
  measures "d780" diameter of A80
  measures "d781" diameter of A79
  measures "d782" diameter of A81
  measures "d783" diameter of A82
  measures "d784" distance between parallel lines of L52 L49
  measures "d785" diameter of A84
  measures "d786" diameter of A85
  measures "d787" diameter of A86
  measures "d788" diameter of A87
  measures "d789" distance of A77.centre point (-105.998, 19.434)
  measures "d790" distance of point (0, 0) point (-101.84, -75.458)
  measures "d791" diameter of A88
  measures "d792" radial gap between concentric circles of A90 A88
  measures "d793" angle of L56 L55
  measures "d794" diameter of A91
  measures "d795" diameter of A92
  measures "d796" distance of L57.start L57.end
  measures "d797" distance of A94.centre A91.centre
  measures "d798" distance of point (-101.84, -75.458) A92.centre
  measures "d799" distance of L61.start L61.end
  measures "d800" vertical distance of L63.start A90.end
  measures "d802" angle of L64 L60
  measures "d803" distance of point (-105.998, 19.434) L65.start
  measures "d804" diameter of A93
  measures "d805" distance between parallel lines of L66 L67
  measures "d806" distance from line of A90.end L67
  measures "d807" distance of L70.end L71.end
  measures "d808" distance of L69.end L70.end
  measures "d809" distance of L74.start A95.centre
  measures "d810" horizontal distance of A88.centre point (-35.56, -322.262)
  measures "d811" distance from line of L66 L64.end
  measures "d812" distance from line of L66 L60.end
  measures "d813" distance of L78.start L78.end
  measures "d814" distance of L77.start L77.end
  measures "d815" distance of A98.centre L63.end
  measures "d816" distance from line of L67 point (0, 0)
  measures "d817" distance from line of L66 L55.start
  measures "d818" distance of L79.start L79.end
  measures "d819" diameter of A100
extrude "Extrusion16" cut sketch "Sketch26" against normal through all contours L41 A87 A43 | A43 A87 L41 | L38 L27 A87 L28 | L28 L33 A82 L47 L27 L38 | A87 A43 L33 L28 L35 | L35 A43 A87 | A87 L27 L28 | L34 A87 A43 | A87 A43 L41 | L41 A43 L33 A87 | A87 L33 A43 | A87 L34 L41 A43 | L41 L34 L28 L33 A43 | L41 L28 A87 L29 | L29 L46 A82 L33 L28 L41 | A87 L28 L29 | L47 A82 L62 L30 L39 L27 | L39 L30 A87 L27 | A87 L30 L27 | L40 L30 L26 A82 L46 L29 | L29 A87 L30 L40 | L29 L30 A87 | L39 L26 A87 A44 | A44 L26 L39 | A82 L33 A85 L62 | A44 A87 L39 L26 | A87 A44 L37 | L37 L39 A44 A87 | A82 L26 A85 L33 | A44 A87 L36 | L39 A87 L26 | A87 A44 L26 L30 L36 | L62 A85 L26 A82 | A82 L26 L30 L62 | L37 L30 L26 A44 L39 | A44 L39 A87 | A85 L26 A83 L33 | L33 A83 L62 A85 | A87 L26 A44 | L39 A44 L26 A87 | L62 A83 L26 A85 | A83 L50 L33 | L33 L50 A83 | L62 L53 L26 A83 | A83 L53 L62 | L50 L51 L52 L53 L26 L33 | L33 L62 L53 L48 L49 L50 | A83 L51 | L49 A83 | L26 L53 A83 | A83 L48 | L62 L26 L53 | A83 L52
fillet "Fillet6" radius 4.7625 4 edges at (-1.5875, 36.8965, 126.6353) (-1.5875, 36.8965, 85.3603) (-1.5875, 1.9715, 85.3603) (-1.5875, 1.9715, 126.6353)